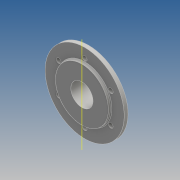
# Autodesk Inventor part: part
Saved by Autodesk Inventor 2016 (Build 200138000, 138)
## iProperties
Created: 2017-09-17
Part Number: part
Material: Generic
Document SubType Name: Modeling
Designer: Fauszt
Density: 1 g/cm^3
Appearance: Default
Author: Fauszt
Autodesk Inventor part; units mm, degrees
ref_plane "YZ Plane" through (0, 0, 0) normal (1, 0, 0) x (0, 1, 0)
ref_plane "XZ Plane" through (0, 0, 0) normal (0, 1, 0) x (-1, 0, 0)
ref_plane "XY Plane" through (0, 0, 0) normal (0, 0, 1) x (1, 0, 0)
sketch "Sketch1" plane through (0, 0, 0) normal (1, 0, 0) x (0, 1, 0)
  line L0 (-2.0441, 0) -> (12.2648, 0) projected
  line L1 (0, -5) -> (0, 30) construction
  line L2 (10.2207, 7.0311) -> (0, 7.0311)
  line L3 (0, 7.0311) -> (0, 25)
  line L4 (0, 25) -> (4.1416, 25)
  line L5 (4.1416, 25) -> (4.1416, 12.8096)
  line L6 (4.1416, 12.8096) -> (10.2207, 12.8096)
  line L7 (10.2207, 12.8096) -> (10.2207, 7.0311)
  point P0 (0, 0)
  dimension "d0" = 50
  constraints: 12 end point, 4 perpendicular, 2 point on line, 1 vertical
  measures "d0" diameter of L4 L0
revolve "Revolution1" add sketch "Sketch1" angle 360 about axis through (0, 0, 0) along (0, 1, 0)
sketch "Sketch2" plane through (0, 0, 0) normal (1, 0, 0) x (0, 1, 0)
  line L0 (0, -35) -> (0, 35) construction
  line L1 (0, 25) -> (4.1416, 25) construction
  line L2 (1.7457, 25) -> (1.7457, 16.7107)
  line L3 (1.7457, 16.7107) -> (0, 16.7107)
  line L4 (-0.8283, 0) -> (4.9699, 0) projected
  line L5 (1.7457, 25) -> (0, 25)
  line L6 (0, -25) -> (0, 25) projected
  line L7 (0, 25) -> (0, 16.7107)
  point P0 (0, 0)
  constraints: 8 end point, 2 horizontal, 2 point on line, 1 collinear, 1 vertical
revolve "Revolution2" cut sketch "Sketch2" angle 360 about axis through (0, -10, 0) along (0, 1, 0)
sketch "Sketch5" plane through (0, 4.1416, 0) normal (0, 1, 0) x (1, 0, 0)
  line L0 (0, 35) -> (0, -35) construction
  point P0 (0, 0)
  point P1 (0, -19)
  dimension "d24" = 19
  constraints: 1 point on line
  measures "d24" distance of point (0, -19) point (0, 0)
hole "Hole3" at (0, 4.1416, 19) direction (0, -1, 0) diameter 3 end through all
pattern_circular "Circular Pattern1" count 6 over 360 about axis through (0, -10, 0) along (0, 1, 0) of "Hole3"
sketch "Sketch6" plane through (0, 0, 0) normal (0, 0, 1) x (1, 0, 0)
  line L0 (25, 4.1416) -> (-25, 4.1416) construction
  line L1 (-12.8096, 4.1416) -> (-12.8096, 10.2207) construction
  line L2 (-12.8096, 4.1416) -> (-12.8096, 8.1416)
  line L3 (-12.8096, 8.1416) -> (-14.8096, 4.1416)
  line L4 (12.8096, 4.1416) -> (-12.8096, 4.1416) projected
  line L5 (-12.8096, 4.1416) -> (-14.8096, 4.1416)
  line L6 (0, -2.0441) -> (0, 12.2648) projected
  point P0 (0, 0)
  dimension "d35" = 2
  dimension "d36" = 4
  constraints: 6 end point, 2 point on line, 1 collinear
  measures "d35" distance of L1.start L3.end
  measures "d36" distance of L1.start L2.end
revolve "Revolution3" add sketch "Sketch6" angle 360 about axis through (0, -10, 0) along (0, 1, 0)
chamfer "Chamfer2" distance 0.5 angle 45 1 edges at (0, 10.2207, -12.8096)
chamfer "Chamfer3" distance 0.5 angle 45 1 edges at (0, 1.7457, -16.7107)
body "Solid1"
